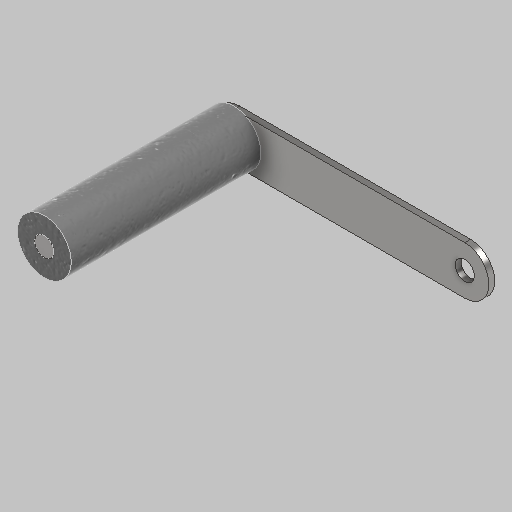
# Autodesk Inventor part: Batente limitador
Saved by Autodesk Inventor 2025.2 (Build 292293000, 293)
## iProperties
Created: 2024-05-02
Part Number: Batente limitador
Material: Genérico
Document SubType Name: Modeling
Designer: phmca
Density: 1 g/cm^3
Appearance: Padrão
Author: phmca
Autodesk Inventor part; units mm, degrees
ref_plane "YZ Plane" through (0, 0, 0) normal (1, 0, 0) x (0, 1, 0)
ref_plane "XZ Plane" through (0, 0, 0) normal (0, 1, 0) x (-1, 0, 0)
ref_plane "XY Plane" through (0, 0, 0) normal (0, 0, 1) x (1, 0, 0)
sketch "Esboço1" plane through (0, 0, 0) normal (0, 0, 1) x (1, 0, 0)
  line L0 (-60, 0) -> (60, 0) construction
  line L1 (-60, -12.5) -> (60, -12.5)
  line L2 (60, 12.5) -> (-60, 12.5)
  arc A0 (-60, 12.5) -> (-60, -12.5) centre (-60, 0) ccw
  arc A1 (60, -12.5) -> (60, 12.5) centre (60, 0) ccw
  circle A2 centre (60, 0) radius 5
  circle A3 centre (-60, 0) radius 5
  point P0 (0, 0)
  dimension "d0" = 25
  dimension "d1" = 10
  dimension "d2" = 10
  dimension "d9" = 120
  constraints: 8 end point, 4 centre point, 4 point on circle, 4 tangent, 2 coincident, 1 horizontal, 1 midpoint, 1 parallel
  measures "d0" distance between parallel lines of L1 L2
  measures "d1" diameter of A2
  measures "d2" diameter of A3
  measures "d9" distance of L0.end L0.start
extrude "Extrusão1" add sketch "Esboço1" along normal mid plane 3 contours A0 L2 A1 L1 | A3
extrude "Extrusão2" add sketch "Esboço1" along normal blind 100 contours A3
sketch "Esboço2" plane through (-60, 0, 100) normal (0, 0, 1) x (1, 0, 0)
  circle A0 centre (0, 0) radius 14
  circle A1 centre (0, 0) radius 5 projected
  point P0 (60, 0)
  dimension "d7" = 100
  dimension "d10" = 28
  dimension "d11" = 10
  constraints: 1 centre point
  measures "d10" diameter of A0
  measures "d11" diameter of A1
extrude "Extrusão3" add sketch "Esboço2" against normal up to surface (98.5 mm away) separate body
